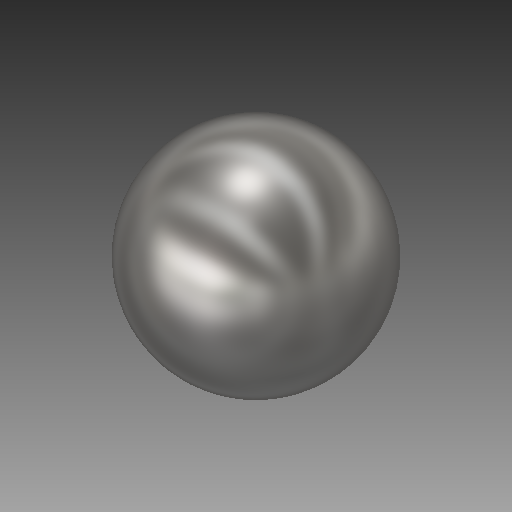
# Autodesk Inventor part: ball bearing ball 0.25in
Saved by Autodesk Inventor 2018 (Build 220112000, 112)
## iProperties
Created: 2017-11-23
Part Number: ball bearing ball 0.25in
Material: Stainless Steel
Document SubType Name: Modeling
Designer: prakh
Density: 8 g/cm^3
Appearance: Semi-Polished
Author: prakh
Autodesk Inventor part; units mm, degrees
ref_plane "YZ Plane" through (0, 0, 0) normal (1, 0, 0) x (0, 1, 0)
ref_plane "XZ Plane" through (0, 0, 0) normal (0, 1, 0) x (-1, 0, 0)
ref_plane "XY Plane" through (0, 0, 0) normal (0, 0, 1) x (1, 0, 0)
sketch "Sketch1" plane through (0, 0, 0) normal (0, 0, 1) x (1, 0, 0)
  arc A0 (0, -3.175) -> (0, 3.175) centre (0, 0) ccw
  line L0 (0, 0) -> (0, 6.3506)
  line L1 (0, 0) -> (0, -9.9461)
  dimension "d0" = 6.35
  constraints: 4 end point, 2 point on circle, 2 point on line, 2 vertical, 1 centre point, 1 coincident
  measures "d0" diameter of A0
revolve "Revolution1" add sketch "Sketch1" angle 360 about axis through (0, 0, 0) along (0, 1, 0)
body "Solid1"
